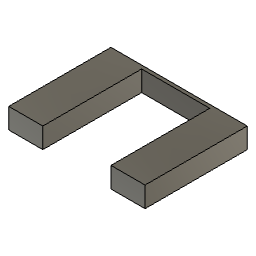
Untitled (Autodesk Fusion 360 design; units mm, degrees)
Autodesk Fusion 360 part; units mm, degrees
sketch "Sketch1" plane through (0, 0, 0) normal (0, 0, 1) x (1, 0, 0)
  line L0 (-2, -15) -> (3, -15)
  line L1 (3, -15) -> (3, 0)
  line L2 (3, 0) -> (-2, 0)
  line L3 (-2, 0) -> (-2, -15)
  line L4 (3, 0) -> (13, 0)
  line L5 (13, 0) -> (13, -0.5)
  line L6 (13, -0.5) -> (3, -0.5)
  line L7 (3, -0.5) -> (3, 0)
  line L8 (13, 0) -> (18, 0)
  line L9 (18, 0) -> (18, -15)
  line L10 (18, -15) -> (13, -15)
  line L11 (13, -15) -> (13, 0)
  dimension "d1" = 5
  dimension "d2" = 15
  dimension "d3" = 10
  dimension "d4" = 0.5
  constraint horizontal L0
  constraint vertical L1
  constraint horizontal L2
  constraint vertical L3
  constraint horizontal L4
  constraint vertical L5
  constraint horizontal L6
  constraint vertical L7
  constraint horizontal L8
  constraint vertical L9
  constraint horizontal L10
  constraint vertical L11
  measures "d1" distance of L0.start L0.end
  measures "d2" distance of L0.start L2.end
  measures "d3" distance of L1.end L4.end
  measures "d4" distance of L1.end L6.end
extrude "Extrude1" add sketch "Sketch1" along normal blind 3
